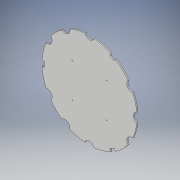
# Autodesk Inventor part: Napduoi
Saved by Autodesk Inventor 2019 (Build 230136000, 136)
## iProperties
Created: 2021-01-20
Part Number: Napduoi
Material: Generic
Document SubType Name: Modeling
Designer: Admin
Density: 1 g/cm^3
Appearance: Default
Author: Admin
Autodesk Inventor part; units mm, degrees
ref_plane "YZ Plane" through (0, 0, 0) normal (1, 0, 0) x (0, 1, 0)
ref_plane "XZ Plane" through (0, 0, 0) normal (0, 1, 0) x (-1, 0, 0)
ref_plane "XY Plane" through (0, 0, 0) normal (0, 0, 1) x (1, 0, 0)
sketch "Sketch1" plane through (0, 0, 0) normal (0, 0, 1) x (1, 0, 0)
  arc A0 (-19.0983, 194.0625) -> (19.0983, 194.0625) centre (0, 200) ccw
  arc A1 (-113.5709, 158.5139) -> (-80.4916, 177.6122) centre (-100, 173.2051) ccw
  arc A2 (-177.6122, 80.4916) -> (-158.5139, 113.5709) centre (-173.2051, 100) ccw
  arc A3 (-194.0625, -19.0983) -> (-194.0625, 19.0983) centre (-200, 0) ccw
  arc A4 (-158.5139, -113.5709) -> (-177.6122, -80.4916) centre (-173.2051, -100) ccw
  arc A5 (-80.4916, -177.6122) -> (-113.5709, -158.5139) centre (-100, -173.2051) ccw
  arc A6 (19.0983, -194.0625) -> (-19.0983, -194.0625) centre (0, -200) ccw
  arc A7 (113.5709, -158.5139) -> (80.4916, -177.6122) centre (100, -173.2051) ccw
  arc A8 (177.6122, -80.4916) -> (158.5139, -113.5709) centre (173.2051, -100) ccw
  arc A9 (194.0625, 19.0983) -> (194.0625, -19.0983) centre (200, 0) ccw
  arc A10 (158.5139, 113.5709) -> (177.6122, 80.4916) centre (173.2051, 100) ccw
  arc A11 (80.4916, 177.6122) -> (113.5709, 158.5139) centre (100, 173.2051) ccw
  arc A12 (-113.5709, 158.5139) -> (-158.5139, 113.5709) centre (0, 0) ccw
  arc A13 (-19.0983, 194.0625) -> (-80.4916, 177.6122) centre (0, 0) ccw
  arc A14 (158.5139, 113.5709) -> (19.0983, 194.0625) centre (0, 0) ccw
  arc A15 (194.0625, 19.0983) -> (177.6122, 80.4916) centre (0, 0) ccw
  arc A16 (177.6122, -80.4916) -> (194.0625, -19.0983) centre (0, 0) ccw
  arc A17 (19.0983, -194.0625) -> (158.5139, -113.5709) centre (0, 0) ccw
  arc A18 (-80.4916, -177.6122) -> (-19.0983, -194.0625) centre (0, 0) ccw
  arc A19 (-177.6122, 80.4916) -> (-177.6122, -80.4916) centre (0, 0) ccw
  arc A20 (-158.5139, -113.5709) -> (-113.5709, -158.5139) centre (0, 0) ccw
  line L0 (0, 0) -> (100, 0) construction
  circle A21 centre (70.7107, 70.7107) radius 1.5
  circle A22 centre (-70.7107, 70.7107) radius 1.5
  circle A23 centre (-70.7107, -70.7107) radius 1.5
  circle A24 centre (70.7107, -70.7107) radius 1.5
  dimension "d2" = 40
  dimension "d5" = 360
  dimension "d9" = 3
  dimension "d12" = 360
  constraints: 42 point on circle, 25 centre point, 2 end point, 1 coincident, 1 horizontal, 58 other
  measures "d2" diameter of A0
  measures "d9" diameter of A21
extrude "Extrusion1" add sketch "Sketch1" along normal blind 5
sketch "Sketch2" plane through (0, 0, 5) normal (0, 0, 1) x (1, 0, 0)
  line L0 (0, 195) -> (10, 195)
  line L1 (10, 195) -> (10, 185)
  line L2 (10, 185) -> (0, 185)
  line L3 (0, 195) -> (-10, 195)
  line L4 (-10, 195) -> (-10, 185)
  line L5 (-10, 185) -> (0, 185)
  line L6 (-106.1603, 163.875) -> (-101.1603, 155.2147)
  line L7 (-97.5, 168.875) -> (-106.1603, 163.875)
  line L8 (-97.5, 168.875) -> (-88.8397, 173.875)
  line L9 (-88.8397, 173.875) -> (-83.8397, 165.2147)
  line L10 (-83.8397, 165.2147) -> (-92.5, 160.2147)
  line L11 (-101.1603, 155.2147) -> (-92.5, 160.2147)
  line L12 (-173.875, 88.8397) -> (-165.2147, 83.8397)
  line L13 (-168.875, 97.5) -> (-173.875, 88.8397)
  line L14 (-168.875, 97.5) -> (-163.875, 106.1603)
  line L15 (-163.875, 106.1603) -> (-155.2147, 101.1603)
  line L16 (-155.2147, 101.1603) -> (-160.2147, 92.5)
  line L17 (-165.2147, 83.8397) -> (-160.2147, 92.5)
  line L18 (-195, -10) -> (-185, -10)
  line L19 (-195, 0) -> (-195, -10)
  line L20 (-195, 0) -> (-195, 10)
  line L21 (-195, 10) -> (-185, 10)
  line L22 (-185, 10) -> (-185, 0)
  line L23 (-185, -10) -> (-185, 0)
  line L24 (-163.875, -106.1603) -> (-155.2147, -101.1603)
  line L25 (-168.875, -97.5) -> (-163.875, -106.1603)
  line L26 (-168.875, -97.5) -> (-173.875, -88.8397)
  line L27 (-173.875, -88.8397) -> (-165.2147, -83.8397)
  line L28 (-165.2147, -83.8397) -> (-160.2147, -92.5)
  line L29 (-155.2147, -101.1603) -> (-160.2147, -92.5)
  line L30 (-88.8397, -173.875) -> (-83.8397, -165.2147)
  line L31 (-97.5, -168.875) -> (-88.8397, -173.875)
  line L32 (-97.5, -168.875) -> (-106.1603, -163.875)
  line L33 (-106.1603, -163.875) -> (-101.1603, -155.2147)
  line L34 (-101.1603, -155.2147) -> (-92.5, -160.2147)
  line L35 (-83.8397, -165.2147) -> (-92.5, -160.2147)
  line L36 (10, -195) -> (10, -185)
  line L37 (0, -195) -> (10, -195)
  line L38 (0, -195) -> (-10, -195)
  line L39 (-10, -195) -> (-10, -185)
  line L40 (-10, -185) -> (0, -185)
  line L41 (10, -185) -> (0, -185)
  line L42 (106.1603, -163.875) -> (101.1603, -155.2147)
  line L43 (97.5, -168.875) -> (106.1603, -163.875)
  line L44 (97.5, -168.875) -> (88.8397, -173.875)
  line L45 (88.8397, -173.875) -> (83.8397, -165.2147)
  line L46 (83.8397, -165.2147) -> (92.5, -160.2147)
  line L47 (101.1603, -155.2147) -> (92.5, -160.2147)
  line L48 (173.875, -88.8397) -> (165.2147, -83.8397)
  line L49 (168.875, -97.5) -> (173.875, -88.8397)
  line L50 (168.875, -97.5) -> (163.875, -106.1603)
  line L51 (163.875, -106.1603) -> (155.2147, -101.1603)
  line L52 (155.2147, -101.1603) -> (160.2147, -92.5)
  line L53 (165.2147, -83.8397) -> (160.2147, -92.5)
  line L54 (195, 10) -> (185, 10)
  line L55 (195, 0) -> (195, 10)
  line L56 (195, 0) -> (195, -10)
  line L57 (195, -10) -> (185, -10)
  line L58 (185, -10) -> (185, 0)
  line L59 (185, 10) -> (185, 0)
  line L60 (163.875, 106.1603) -> (155.2147, 101.1603)
  line L61 (168.875, 97.5) -> (163.875, 106.1603)
  line L62 (168.875, 97.5) -> (173.875, 88.8397)
  line L63 (173.875, 88.8397) -> (165.2147, 83.8397)
  line L64 (165.2147, 83.8397) -> (160.2147, 92.5)
  line L65 (155.2147, 101.1603) -> (160.2147, 92.5)
  line L66 (88.8397, 173.875) -> (83.8397, 165.2147)
  line L67 (97.5, 168.875) -> (88.8397, 173.875)
  line L68 (97.5, 168.875) -> (106.1603, 163.875)
  line L69 (106.1603, 163.875) -> (101.1603, 155.2147)
  line L70 (101.1603, 155.2147) -> (92.5, 160.2147)
  line L71 (83.8397, 165.2147) -> (92.5, 160.2147)
  point P0 (0, 0)
  point P1 (0, 0)
  dimension "d17" = 10
  dimension "d18" = 10
  dimension "d21" = 360
  constraints: 144 end point, 1 coincident, 1 horizontal, 1 parallel, 1 perpendicular, 145 other
  measures "d17" distance of L1.end L2.end
  measures "d18" distance of L0.end L1.end
extrude "Extrusion2" cut sketch "Sketch2" against normal blind 5 contours L19 L20 L21 L22 L23 L18 | L43 L44 L45 L46 L47 L42 | L67 L68 L69 L70 L71 L66
body "Solid1"
